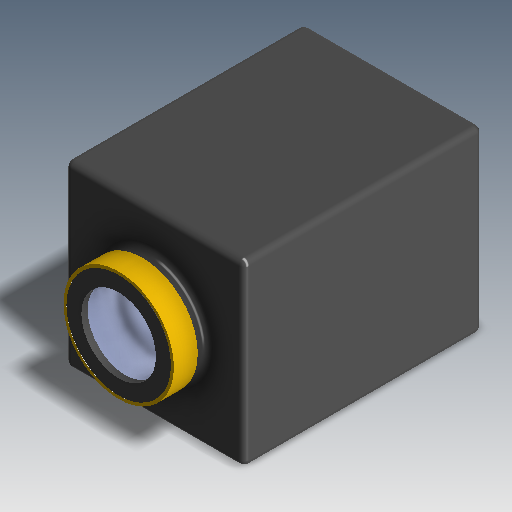
# Autodesk Inventor part: Power Meter
Saved by Autodesk Inventor 2026 (Build 300175050, 175E)
## iProperties
Created: 2025-08-02
Part Number: Power Meter
Material: Generic
Document SubType Name: Modeling
Designer: aman0
Density: 1 g/cm^3
Appearance: Default
Author: aman0
Autodesk Inventor part; units mm, degrees
ref_plane "YZ Plane" through (0, 0, 0) normal (1, 0, 0) x (0, 1, 0)
ref_plane "XZ Plane" through (0, 0, 0) normal (0, 1, 0) x (-1, 0, 0)
ref_plane "XY Plane" through (0, 0, 0) normal (0, 0, 1) x (1, 0, 0)
sketch "Sketch5" plane through (0, 0, 0) normal (0, 1, 0) x (-1, 0, 0)
  line L0 (0, 0) -> (0, 2)
  circle A0 centre (0, -38.0625) radius 40.0625
  line L1 (0, 0) -> (12.5, 0)
  line L2 (0, 0) -> (-12.5, 0)
  dimension "d31" = 2
  dimension "d32" = 12.5
  dimension "d33" = 12.5
  constraints: 6 end point, 3 point on circle, 1 centre point, 1 horizontal, 1 point on line, 1 vertical
  measures "d31" distance of L0.start L0.end
  measures "d32" distance of L0.start L1.end
  measures "d33" distance of L0.start L2.end
revolve "Revolution1" add sketch "Sketch5" angle 360 about axis through (0, 0, 0) along (0, 0, 1) contours L2 A0 L0
sketch "Sketch6" plane through (0, 0, 0) normal (0, 0, -1) x (-1, 0, 0)
  circle A0 centre (0, 0) radius 12.5
  circle A1 centre (0, 0) radius 17.5
  dimension "d35" = 25
  dimension "d36" = 35
  constraints: 2 centre point, 2 coincident
  measures "d35" diameter of A0
  measures "d36" diameter of A1
extrude "Extrusion5" add sketch "Sketch6" along normal blind 10 and the other way blind 2
sketch "Sketch7" plane through (0, 0, -10) normal (0, 0, -1) x (-1, 0, 0)
  line L0 (-30, -30) -> (30, -30)
  line L1 (30, -30) -> (30, 30)
  line L2 (30, 30) -> (-30, 30)
  line L3 (-30, 30) -> (-30, -30)
  line L4 (-30, -30) -> (30, 30) construction
  line L5 (30, -30) -> (-30, 30) construction
  point P0 (0, 0)
  dimension "d41" = 60
  dimension "d42" = 60
  constraints: 12 end point, 2 midpoint, 2 parallel, 1 horizontal, 1 perpendicular
  measures "d41" distance of L0.start L0.end
  measures "d42" distance of L1.end L0.end
extrude "Extrusion6" add sketch "Sketch7" along normal blind 80
fillet "Fillet1" radius 2 13 edges at (0, 30, -10) (30, 0, -10) (30, 30, -50) (30, 0, -90) (30, -30, -50) (0, 30, -90) (-30, 30, -50) (-30, 0, -10) (17.5, 0, -10) (0, -30, -10) (-30, -30, -50) (0, -30, -90) (-30, 0, -90)
sketch "Sketch8" plane through (0, 0, 2) normal (0, 0, 1) x (1, 0, 0)
  circle A0 centre (0, 0) radius 17.505
  circle A1 centre (0, 0) radius 18.5
  dimension "d46" = 35.01
  dimension "d47" = 37
  constraints: 2 centre point, 2 coincident
  measures "d46" diameter of A0
  measures "d47" diameter of A1
extrude "Extrusion7" add sketch "Sketch8" against normal blind 8
body "Solid2"
